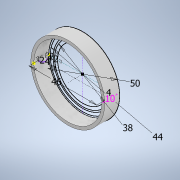
# Autodesk Inventor part: probe_gimbal_prototype
Saved by Autodesk Inventor 2021 (Build 250183000, 183)
## iProperties
Created: 2021-06-06
Part Number: probe_gimbal_prototype
Material: Generic
Document SubType Name: Modeling
Designer: Charlie
Density: 1 g/cm^3
Appearance: Default
Author: Charlie
Autodesk Inventor part; units mm, degrees
ref_plane "YZ Plane" through (0, 0, 0) normal (1, 0, 0) x (0, 1, 0)
ref_plane "XZ Plane" through (0, 0, 0) normal (0, 1, 0) x (-1, 0, 0)
ref_plane "XY Plane" through (0, 0, 0) normal (0, 0, 1) x (1, 0, 0)
sketch "Sketch1" plane through (0, 0, 0) normal (0, 0, 1) x (1, 0, 0)
  circle A0 centre (0, 0) radius 25
  circle A1 centre (0, 0) radius 23
  circle A2 centre (0, 0) radius 22
  circle A3 centre (0, 0) radius 20
  circle A4 centre (0, 0) radius 19
  circle A5 centre (0, 0) radius 17
  line L0 (25, 0) -> (-25, 0) construction
  line L1 (0, 25) -> (0, -25) construction
  dimension "d0" = 50
  dimension "d1" = 2
  dimension "d2" = 44
  dimension "d3" = 2
  dimension "d4" = 38
  dimension "d5" = 2
  constraints: 6 centre point, 4 end point, 4 point on circle, 3 coincident, 1 horizontal, 1 perpendicular
  measures "d0" diameter of A0
  measures "d1" radial gap between concentric circles of A0 A1
  measures "d2" diameter of A2
  measures "d3" radial gap between concentric circles of A2 A3
  measures "d4" diameter of A4
  measures "d5" radial gap between concentric circles of A4 A5
extrude "Extrusion2" add sketch "Sketch1" along normal blind 10 contours A0
sketch "Sketch2" plane through (0, 0, 0) normal (0, 1, 0) x (-1, 0, 0)
  line L0 (-23, 0) -> (23, 0) construction
  line L1 (23, 0) -> (-23, 0) construction
  line L2 (-23, 0) -> (-23, 10) construction
  line L3 (23, 10) -> (23, 0) construction
  line L4 (23, 10) -> (23, 0) construction
  circle A0 centre (23, 5) radius 2 construction
  line L5 (0, 0) -> (0, 10) construction
  circle A1 centre (-23, 5) radius 2 construction
  line L6 (24.0412, 3.2924) -> (23, 7)
  line L7 (-23, 0) -> (-23, 10)
  line L8 (23, 10) -> (23, 0) construction
  line L9 (-23, 5) -> (23, 5) construction
  line L10 (23, 10) -> (23, 0) construction
  circle A2 centre (-22.1677, 5) radius 2
  circle A3 centre (22.2113, 5) radius 2
  line L11 (20.2113, 5) -> (24.2113, 5)
  line L12 (-20.1677, 5) -> (-24.1677, 5)
  point P0 (-23, 7)
  point P1 (-23, 3)
  dimension "d12" = 4
  dimension "d11" = 10
  dimension "d31" = 46
  dimension "d32" = 4
  dimension "d33" = 4
  constraints: 18 end point, 6 point on line, 4 point on circle, 3 centre point, 1 coincident, 1 horizontal, 1 midpoint, 1 parallel, 1 perpendicular, 1 symmetric about line, 1 vertical, 1 vertical alignment, 2 other
  measures "d11" distance of L1.end L2.end
  measures "d31" distance of L9.end L9.start
  measures "d32" diameter of A2
  measures "d33" diameter of A3
revolve "Revolution1" add sketch "Sketch2" angle 360 about axis through (23, 0, 5) along (-1, 0, 0) picked at (21.3446, 5.1473) picked at (23.3511, 6.1311) contours L11 A3 L6 | L6 A3 L11
revolve "Revolution2" add sketch "Sketch2" angle 360 about axis through (23, 0, 5) along (-1, 0, 0) picked at (-23.13, 6.1339) picked at (-21.1282, 5.1469) contours L12 A2 L7 | L7 A2 L12
body "Solid2"
